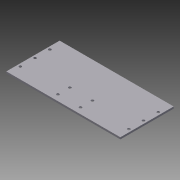
# Autodesk Inventor part: Chassis Back
Saved by Autodesk Inventor 2012 (Build 160160000, 160)
## iProperties
Created: 2012-04-05
Part Number: Chassis Back
Material: Aluminum-6061
Document SubType Name: Modeling
Designer: Jaime
Density: 2.71 g/cm^3
Mass: 151.409 g
Surface Area: 376.109 cm^2
Volume: 55.8705 cm^3
Author: Jaime
Autodesk Inventor part; units mm, degrees
ref_plane "YZ Plane" through (0, 0, 0) normal (1, 0, 0) x (0, 1, 0)
ref_plane "XZ Plane" through (0, 0, 0) normal (0, 1, 0) x (-1, 0, 0)
ref_plane "XY Plane" through (0, 0, 0) normal (0, 0, 1) x (1, 0, 0)
sketch "Sketch1" plane through (0, 0, 0) normal (0, 0, 1) x (1, 0, 0)
  line L0 (0, -10.16) -> (195.58, -10.16)
  line L1 (195.58, -10.16) -> (195.58, -101.6)
  line L2 (195.58, -101.6) -> (0, -101.6)
  line L3 (0, -101.6) -> (0, -10.16)
  point P0 (0, 0)
  dimension "d27" = 91.44
  dimension "d28" = 195.58
  constraints: 8 end point, 2 parallel, 1 horizontal, 1 perpendicular
  measures "d27" distance of L0.end L1.end
  measures "d28" distance of L0.start L0.end
extrude "Extrusion2" add sketch "Sketch1" along normal blind 3.175
sketch "Sketch3" plane through (0, 0, 0) normal (0, 0, -1) x (-1, 0, 0)
  circle A0 centre (-190.8175, -82.296) radius 1.651 projected
  circle A1 centre (-190.8175, -57.15) radius 1.651 projected
  circle A2 centre (-190.8175, -31.75) radius 1.651 projected
  circle A3 centre (-117.1575, -91.44) radius 1.651 projected
  circle A4 centre (-117.1575, -71.12) radius 1.651 projected
  circle A5 centre (-78.4225, -71.12) radius 1.651 projected
  circle A6 centre (-78.4225, -91.44) radius 1.651 projected
  circle A7 centre (-4.7625, -82.296) radius 1.651 projected
  circle A8 centre (-4.7625, -57.15) radius 1.651 projected
  circle A9 centre (-4.7625, -31.75) radius 1.651 projected
  point P0 (0, 0)
  constraints: 10 coincident
hole "Hole2" at (190.8175, -31.75, 0) at (190.8175, -57.15, 0) at (190.8175, -82.296, 0) at (117.1575, -71.12, 0) at (117.1575, -91.44, 0) at (78.4225, -71.12, 0) at (78.4225, -91.44, 0) at (4.7625, -82.296, 0) at (4.7625, -57.15, 0) at (4.7625, -31.75, 0) direction (0, 0, 1) diameter 4.4958 end through all countersink diameter 8.4328 countersink angle 82 clearance for "Flat Head Machine Screw (82)" size "#8" standard "Ansi Unified Screw Threads"
body "Solid2"
